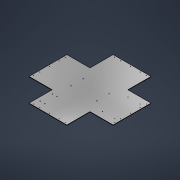
# Autodesk Inventor part: 200510
Saved by Autodesk Inventor 2022.2 (Build 262287000, 287)
## iProperties
Created: 2022-08-10
Part Number: 200510
Material: Aluminum 5052 H32
Document SubType Name: Sheet Metal
Designer: robotics
Density: 2.7 g/cm^3
Sheet Metal Rule: .125 5052
Appearance: Aluminum - Flat
Mass: 2912.99 g
Surface Area: 6899.52 cm^2
Volume: 1078.89 cm^3
GlobalPropertyList: <PropertyList/>
Author: robotics
Autodesk Inventor part; units mm, degrees
ref_plane "YZ Plane" through (0, 0, 0) normal (1, 0, 0) x (0, 1, 0)
ref_plane "XZ Plane" through (0, 0, 0) normal (0, 1, 0) x (-1, 0, 0)
ref_plane "XY Plane" through (0, 0, 0) normal (0, 0, 1) x (1, 0, 0)
sketch "Sketch1" plane through (0, 0, 0) normal (0, 1, 0) x (-1, 0, 0)
  line L0 (0, 0) -> (0, -314.325)
  line L1 (0, -314.325) -> (192.0875, -314.325)
  line L2 (192.0875, -314.325) -> (192.0875, -506.4125)
  line L3 (192.0875, -506.4125) -> (506.4125, -506.4125)
  line L4 (506.4125, -506.4125) -> (506.4125, -314.325)
  line L5 (506.4125, -314.325) -> (698.5, -314.325)
  line L6 (698.5, -314.325) -> (698.5, 0)
  line L7 (698.5, 0) -> (506.4125, 0)
  line L8 (506.4125, 0) -> (506.4125, 192.0875)
  line L9 (506.4125, 192.0875) -> (192.0875, 192.0875)
  line L10 (192.0875, 192.0875) -> (192.0875, 0)
  line L11 (192.0875, 0) -> (0, 0)
  line L12 (698.5, 192.0875) -> (0, 192.0875) construction
  line L13 (0, 192.0875) -> (0, -506.4125) construction
  line L14 (0, -506.4125) -> (698.5, -506.4125) construction
  line L15 (698.5, -506.4125) -> (698.5, 192.0875) construction
  dimension "d0" = 698.5
  dimension "d1" = 192.0875
  measures "d0" distance of L14.end L12.start
  measures "d1" distance of L7.end L8.end
extrude "Plate1" add sketch "Sketch1" along normal blind 3.175
sketch "Sketch2" plane through (0, 3.175, 0) normal (0, 1, 0) x (1, 0, 0)
  line L0 (-506.4125, 506.4125) -> (-192.0875, 506.4125) projected
  line L1 (0, 314.325) -> (0, 0) projected
  line L2 (-192.0875, -192.0875) -> (-506.4125, -192.0875) projected
  line L3 (-698.5, 0) -> (-698.5, 314.325) projected
  line L4 (-506.4125, 314.325) -> (-506.4125, 506.4125) projected
  line L5 (-192.0875, 506.4125) -> (-192.0875, 314.325) projected
  line L6 (-698.5, 314.325) -> (-506.4125, 314.325) projected
  line L7 (-506.4125, 0) -> (-698.5, 0) projected
  line L8 (-349.25, 506.4125) -> (-349.25, -192.0875) construction
  line L9 (-698.5, 157.1625) -> (0, 157.1625) construction
  point P0 (-481.0125, 493.7125)
  point P1 (-430.2125, 493.7125)
  point P2 (-268.2875, 493.7125)
  point P3 (-217.4875, 493.7125)
  point P4 (-12.7, 288.925)
  point P5 (-12.7, 238.125)
  point P6 (-12.7, 76.2)
  point P7 (-12.7, 25.4)
  point P8 (-217.4875, -179.3875)
  point P9 (-268.2875, -179.3875)
  point P10 (-430.2125, -179.3875)
  point P11 (-481.0125, -179.3875)
  point P12 (-685.8, 25.4)
  point P13 (-685.8, 76.2)
  point P14 (-685.8, 238.125)
  point P15 (-685.8, 288.925)
  point P16 (-349.25, 493.7125)
  point P17 (-349.25, -179.3875)
  point P18 (-685.8, 157.1625)
  point P19 (-12.7, 157.1625)
  dimension "d3" = 12.7
  dimension "d4" = 12.7
  dimension "d5" = 12.7
  dimension "d6" = 12.7
  dimension "d7" = 25.4
  dimension "d8" = 50.8
  dimension "d9" = 25.4
  dimension "d10" = 50.8
  dimension "d11" = 25.4
  dimension "d12" = 50.8
  dimension "d13" = 25.4
  dimension "d14" = 50.8
  constraints: 12 horizontal alignment, 12 vertical alignment, 4 end point, 4 midpoint, 4 point on line
  measures "d3" distance from line of L0 point (-481.012, 493.712)
  measures "d4" distance from line of L1 point (-12.7, 288.925)
  measures "d5" distance from line of L2 point (-217.488, -179.388)
  measures "d6" distance from line of L3 point (-685.8, 288.925)
  measures "d7" distance from line of L4 point (-481.012, 493.712)
  measures "d8" distance of point (-430.212, 493.712) point (-481.012, 493.712)
  measures "d9" distance from line of L5 point (-217.488, 493.712)
  measures "d10" distance of point (-268.288, 493.712) point (-217.488, 493.712)
  measures "d11" distance from line of L6 point (-685.8, 288.925)
  measures "d12" distance of point (-685.8, 288.925) point (-685.8, 238.125)
  measures "d13" distance from line of L7 point (-685.8, 25.4)
  measures "d14" distance of point (-685.8, 76.2) point (-685.8, 25.4)
hole "Hole1" at (-685.8, 3.175, -288.925) at (-685.8, 3.175, -238.125) at (-685.8, 3.175, -76.2) at (-685.8, 3.175, -25.4) at (-481.0125, 3.175, 179.3875) at (-430.2125, 3.175, 179.3875) at (-268.2875, 3.175, 179.3875) at (-217.4875, 3.175, 179.3875) at (-12.7, 3.175, -25.4) at (-12.7, 3.175, -76.2) at (-12.7, 3.175, -238.125) at (-12.7, 3.175, -288.925) at (-217.4875, 3.175, -493.7125) at (-268.2875, 3.175, -493.7125) at (-430.2125, 3.175, -493.7125) at (-481.0125, 3.175, -493.7125) at (-685.8, 3.175, -157.1625) at (-349.25, 3.175, 179.3875) at (-12.7, 3.175, -157.1625) at (-349.25, 3.175, -493.7125) direction (0, -1, 0) diameter 4.0894 end through all clearance for "Pop Rivet" size "5/32" standard "4859 Fastners"
sketch "Sketch3" plane through (0, 3.175, 0) normal (0, 1, 0) x (1, 0, 0)
  circle A0 centre (-12.7, 25.4) radius 2.0447 construction
sketch "Sketch4" plane through (0, 3.175, 0) normal (0, 1, 0) x (1, 0, 0)
  circle A0 centre (-12.7, 76.2) radius 2.0447 construction
sketch "Sketch5" plane through (0, 3.175, 0) normal (0, 1, 0) x (1, 0, 0)
  circle A0 centre (-456.9079, 207.9586) radius 2.5 projected
  circle A1 centre (-241.0079, 207.9586) radius 2.5 projected
  circle A2 centre (-241.0079, 106.3586) radius 2.5 projected
  circle A3 centre (-456.9079, 106.3586) radius 2.5 projected
  point P0 (0, 0)
hole "Hole2" at (-456.9079, 3.175, -207.9586) at (-241.0079, 3.175, -207.9586) at (-456.9079, 3.175, -106.3586) at (-241.0079, 3.175, -106.3586) direction (0, -1, 0) diameter 5.1054 end through all clearance for "Socket Head Cap Screw" size "#10" standard "4859 Fastners"
sketch "Sketch6" plane through (0, 3.175, 0) normal (0, 1, 0) x (1, 0, 0)
  circle A0 centre (-475.0703, -29.3212) radius 2.5 projected
  circle A1 centre (-436.9703, -29.3212) radius 2.5 projected
  circle A2 centre (-475.0703, -130.9212) radius 2.5 projected
  circle A3 centre (-436.9703, -130.9212) radius 2.5 projected
  point P0 (0, 0)
hole "Hole3" at (-475.0703, 3.175, 130.9212) at (-436.9703, 3.175, 130.9212) at (-475.0703, 3.175, 29.3212) at (-436.9703, 3.175, 29.3212) direction (0, -1, 0) diameter 5.1054 end through all clearance for "Socket Head Cap Screw" size "#10" standard "4859 Fastners"
sketch "Sketch8" plane through (0, 3.175, 0) normal (0, 1, 0) x (1, 0, 0)
  circle A0 centre (-139.7, 262.7312) radius 2.0447 projected
  circle A1 centre (-38.1, 262.7312) radius 2.0447 projected
  circle A2 centre (-139.7, 51.5937) radius 2.0447 projected
  circle A3 centre (-38.1, 51.5937) radius 2.0447 projected
  circle A4 centre (-209.2008, 207.9625) radius 2.0447 projected
  circle A5 centre (-209.2008, 106.3625) radius 2.0447 projected
  point P0 (0, 0)
hole "Hole4" at (-139.7, 3.175, -262.7312) at (-38.1, 3.175, -262.7312) at (-139.7, 3.175, -51.5937) at (-38.1, 3.175, -51.5937) at (-209.2008, 3.175, -207.9625) at (-209.2008, 3.175, -106.3625) direction (0, -1, 0) diameter 4.0894 end through all clearance for "Pop Rivet" size "5/32" standard "4859 Fastners"
equation "\"d9\" = d7"
equation "\"d10\" = d8"
equation "\"d11\" = d7"
equation "\"d12\" = d8"
equation "\"d13\" = d7"
equation "\"d14\" = d8"
equation "\"d0\" = DrivebaseLength"
equation "\"d1\" = PlateCut"
equation "\"d20\" = Thickness"
equation "\"d27\" = Thickness"
equation "\"d41\" = Thickness"
equation "\"d2\" = Thickness"
equation "\"BendRadius\" = 1.5 * Thickness"
equation "\"BendReliefWidth\" = Thickness"
equation "\"BendReliefDepth\" = 0.5 * Thickness"
equation "\"CornerReliefSize\" = 4 * Thickness"
equation "\"MinimumRemnant\" = 2 * Thickness"
equation "\"TransitionRadius\" = BendRadius"
equation "\"JacobiRadiusSize\" = BendRadius"
equation "\"GapSize\" = Thickness"
equation "\"DrivebaseLength\" = 698.5"
equation "\"DrivebaseWidth\" = 698.5"
equation "\"LengthOfTube\" = 482.6"
equation "\"ModuleSize\" = 169.8625"
equation "\"EdgeModuleToHole\" = 61.9125"
equation "\"ModuleSpace\" = 107.95"
equation "\"HoleLength1\" = 6.35"
equation "\"HoleLength2\" = 31.75"
equation "\"HoleLength3\" = 57.15"
equation "\"HoleLength4\" = 425.45"
equation "\"HoleLength5\" = 450.85"
equation "\"HoleLength6\" = 476.25"
equation "\"HoleWidth\" = 12.7"
equation "\"ModuleLength\" = 190.5"
equation "\"PlateCut\" = 192.0875"
equation "\"Rivet1\" = 109.5375"
equation "\"Rivet2\" = 160.3375"
equation "\"Rivet4\" = 322.2625"
equation "\"Rivet3\" = 241.3"
equation "\"Rivet5\" = 373.0625"
equation "\"Thickness\" = 3.175"
body "Solid1"
